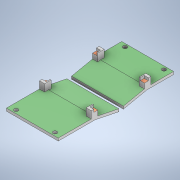
# Autodesk Inventor part: air_duct_inside
Saved by Autodesk Inventor 2022 (Build 260153000, 153)
## iProperties
Created: 2022-10-27
Part Number: air_duct_inside
Material: Ogólny
Document SubType Name: Modeling
Designer: kosak
Density: 1 g/cm^3
Appearance: Domyślna
Author: kosak
Autodesk Inventor part; units mm, degrees
ref_plane "YZ Plane" through (0, 0, 0) normal (1, 0, 0) x (0, 1, 0)
ref_plane "XZ Plane" through (0, 0, 0) normal (0, 1, 0) x (-1, 0, 0)
ref_plane "XY Plane" through (0, 0, 0) normal (0, 0, 1) x (1, 0, 0)
sketch "Szkic1" plane through (0, 0, 0) normal (0, 1, 0) x (-1, 0, 0)
  line L0 (0, 0) -> (40, 0)
  line L1 (40, 0) -> (40, -28.5)
  line L2 (40, -28.5) -> (0, -28.5)
  line L3 (0, -28.5) -> (0, 0)
  line L4 (0, -68.5) -> (40, -68.5)
  line L5 (40, -68.5) -> (40, -89)
  line L6 (40, -89) -> (0, -89)
  line L7 (0, -89) -> (0, -68.5)
  line L8 (22.9187, -28.5) -> (22.9187, -68.5)
  dimension "d0" = 40
  dimension "d1" = 28.5
  dimension "d3" = 20.5
  dimension "d84" = 40
  constraints: 18 end point, 4 parallel, 3 perpendicular, 2 horizontal, 2 point on line
  measures "d0" distance of L1.end L2.end
  measures "d1" distance of L0.end L1.end
  measures "d3" distance of L4.end L5.end
  measures "d84" distance of L8.start L8.end
extrude "Wyciągnięcie proste1" add sketch "Szkic1" along normal blind 2
sketch "Szkic2" plane through (0, 0, 0) normal (1, 0, 0) x (0, 0, -1)
  line L0 (48.4992, 0) -> (48.4992, -3.8)
  line L1 (0, 0) -> (28.5, 0) projected
  line L2 (28.5, 0) -> (48.5, 0)
  line L3 (89, 0) -> (68.5, 0) projected
  line L4 (48.4992, -3.8) -> (50.2492, -3.8)
  line L5 (48.4992, -3.8) -> (46.7492, -3.8)
  line L6 (28.5, 0) -> (46.7492, -3.8)
  line L7 (28.5, 0) -> (28.5, 2) projected
  line L8 (28.5, 2) -> (46.7492, -1.8)
  line L9 (46.7492, -1.8) -> (46.7492, -3.8)
  line L10 (68.5, 0) -> (50.2492, -3.8)
  line L11 (68.5, 0) -> (68.5, 2) projected
  line L12 (68.5, 2) -> (50.2492, -1.8)
  line L13 (50.2492, -1.8) -> (50.2492, -3.8)
  dimension "d8" = 20
  constraints: 20 end point, 4 parallel, 2 horizontal, 1 collinear, 1 point on line, 1 vertical
  measures "d8" distance of L1.end L2.end
extrude "Wyciągnięcie proste2" add sketch "Szkic2" against normal blind 40 contours L13 L12 L11 L10 | L8 L9 L6 L2 | L2 L7 L8
sketch "Szkic3" plane through (0, 2, 0) normal (0, 1, 0) x (1, 0, 0)
  line L0 (-40, 46.7492) -> (-40, 28.5) projected
  line L1 (-40, 28.5) -> (-36, 28.5)
  line L2 (-36, 28.5) -> (-36, 25.5)
  line L3 (-36, 25.5) -> (-40, 25.5)
  line L4 (-40, 25.5) -> (-40, 28.5)
  line L5 (-36, 28.5) -> (-40, 28.5)
  line L6 (-40, 28.5) -> (-40, 30.5)
  line L7 (-40, 30.5) -> (-36, 30.5)
  line L8 (-36, 30.5) -> (-36, 28.5)
  line L9 (-36, 71.5) -> (-36, 69.5)
  line L10 (-40, 71.5) -> (-36, 71.5)
  line L11 (-40, 69.5) -> (-40, 71.5)
  line L12 (-40, 66.5) -> (-40, 69.5)
  line L13 (-36, 66.5) -> (-40, 66.5)
  line L14 (-36, 69.5) -> (-36, 66.5)
  line L15 (0, 28.5) -> (0, 25.5)
  line L16 (0, 30.5) -> (0, 28.5)
  line L17 (-4, 30.5) -> (0, 30.5)
  line L18 (-4, 28.5) -> (-4, 30.5)
  line L19 (-4, 25.5) -> (-4, 28.5)
  line L20 (0, 25.5) -> (-4, 25.5)
  line L21 (-4, 71.5) -> (0, 71.5)
  line L22 (-4, 69.5) -> (-4, 71.5)
  line L23 (-4, 66.5) -> (-4, 69.5)
  line L24 (0, 69.5) -> (0, 66.5)
  line L25 (0, 71.5) -> (0, 69.5)
  line L26 (0, 66.5) -> (-4, 66.5)
  point P0 (0, 0)
  dimension "d13" = 4
  dimension "d14" = 3
  dimension "d15" = 2
  dimension "d18" = 41
  dimension "d25" = 36
  dimension "d32" = 36
  constraints: 52 end point, 4 horizontal, 4 parallel, 3 collinear, 2 perpendicular, 1 point on line, 1 vertical, 36 other
  measures "d13" distance of L2.end L3.end
  measures "d14" distance of L1.end L2.end
  measures "d15" distance of L5.end L6.end
  measures "d18" distance of L7.end L9.start
  measures "d25" distance of L1.end L15.start
  measures "d32" distance of L10.start L21.start
extrude "Wyciągnięcie proste3" add sketch "Szkic3" along normal blind 3.5
sketch "Szkic5" plane through (-40, 0, -89) normal (-1, 0, 0) x (0, 0, 1)
  line L0 (22.5, 2) -> (20.5, 2) projected
  line L1 (22.5, 2) -> (20.5, 2)
  line L2 (20.5, 2) -> (22.5, 1.5836)
  line L3 (38.7508, -1.8) -> (20.5, 2) projected
  line L4 (20.5, 2) -> (22.5, 2) projected
  line L5 (22.5, 2) -> (22.5, 1.5836)
  line L6 (58.5, 2) -> (60.5, 2) projected
  line L7 (60.5, 2) -> (42.2508, -1.8) projected
  line L8 (60.5, 2) -> (58.5, 2)
  line L9 (58.5, 1.5835) -> (58.5, 2)
  line L10 (58.5, 1.5835) -> (60.5, 2)
  point P0 (89, 0)
  constraints: 12 end point, 3 collinear, 2 perpendicular, 2 point on line
extrude "Wyciągnięcie proste5" add sketch "Szkic5" against normal blind 4
sketch "Szkic6" plane through (0, 5.5, 0) normal (0, 1, 0) x (1, 0, 0)
  line L0 (-36, 25.5) -> (-36, 30.5) projected
  line L1 (-36, 25.5) -> (-40, 25.5) projected
  line L2 (-36, 30.5) -> (-36.8, 30.5)
  line L3 (-36.8, 30.5) -> (-36.8, 25.5)
  line L4 (-36.8, 25.5) -> (-36, 25.5)
  line L5 (-36, 25.5) -> (-36, 30.5)
  line L6 (-36, 66.5) -> (-36, 71.5)
  line L7 (-36.8, 71.5) -> (-36.8, 66.5)
  line L8 (-36.8, 66.5) -> (-36, 66.5)
  line L9 (-36, 71.5) -> (-36.8, 71.5)
  line L10 (-4, 30.5) -> (-4, 25.5)
  line L11 (-3.2, 25.5) -> (-3.2, 30.5)
  line L12 (-3.2, 30.5) -> (-4, 30.5)
  line L13 (-4, 25.5) -> (-3.2, 25.5)
  line L14 (-4, 71.5) -> (-4, 66.5)
  line L15 (-3.2, 66.5) -> (-3.2, 71.5)
  line L16 (-3.2, 71.5) -> (-4, 71.5)
  line L17 (-4, 66.5) -> (-3.2, 66.5)
  point P0 (0, 0)
  dimension "d43" = 0.8
  dimension "d48" = 41
  dimension "d55" = 32.8
  constraints: 32 end point, 2 horizontal, 2 parallel, 1 collinear, 1 perpendicular, 1 point on line, 1 vertical, 24 other
  measures "d43" distance of L4.end L3.end
  measures "d48" distance of L4.end L6.start
  measures "d55" distance of L2.end L10.start
extrude "Wyciągnięcie proste6" add sketch "Szkic6" along normal blind 2
sketch "Szkic7" plane through (0, 5.5, 0) normal (0, 1, 0) x (1, 0, 0)
  line L0 (-40, 25.5) -> (-40, 0) projected
  line L1 (-36.8, 30.5) -> (-36.8, 25.5) projected
  line L2 (-40, 25.5) -> (-36.8, 25.5)
  line L3 (-36.8, 25.5) -> (-36.8, 27.5)
  line L4 (-36.8, 27.5) -> (-40, 27.5)
  line L5 (-40, 27.5) -> (-40, 25.5)
  line L6 (-36.8, 71.5) -> (-40, 71.5)
  line L7 (-40, 71.5) -> (-40, 69.5)
  line L8 (-40, 69.5) -> (-36.8, 69.5)
  line L9 (-36.8, 69.5) -> (-36.8, 71.5)
  line L10 (-3.2, 71.5) -> (-3.2, 69.5)
  line L11 (-3.2, 69.5) -> (0, 69.5)
  line L12 (0, 69.5) -> (0, 71.5)
  line L13 (0, 71.5) -> (-3.2, 71.5)
  line L14 (-3.2, 25.5) -> (0, 25.5)
  line L15 (-3.2, 27.5) -> (-3.2, 25.5)
  line L16 (0, 27.5) -> (-3.2, 27.5)
  line L17 (0, 25.5) -> (0, 27.5)
  point P0 (0, 0)
  dimension "d60" = 2
  dimension "d63" = 44
  dimension "d70" = 36.8
  dimension "d77" = 44
  constraints: 32 end point, 3 collinear, 2 horizontal, 2 parallel, 2 vertical, 1 perpendicular, 1 point on line, 21 other
  measures "d60" distance of L3.end L2.end
  measures "d63" distance of L3.end L6.start
  measures "d70" distance of L6.end L10.start
  measures "d77" distance of L10.end L14.start
extrude "Wyciągnięcie proste7" add sketch "Szkic7" along normal blind 2
sketch "Szkic8" plane through (0, 0, 0) normal (1, 0, 0) x (0, 0, -1)
  line L0 (28.5, 2) -> (30.5, 2) projected
  line L1 (28.5, 2) -> (30.5, 2)
  line L2 (30.5, 2) -> (30.5, 1.5835)
  line L3 (46.7492, -1.8) -> (28.5, 2) projected
  line L4 (28.5, 2) -> (30.5, 1.5835)
  line L5 (66.5, 2) -> (68.5, 2) projected
  line L6 (66.5, 2) -> (68.5, 2)
  line L7 (68.5, 2) -> (50.2492, -1.8) projected
  line L8 (66.5, 2) -> (66.5, 1.5836)
  line L9 (66.5, 1.5836) -> (68.5, 2)
  point P0 (0, 0)
  constraints: 12 end point, 2 collinear, 2 point on line, 1 horizontal, 1 perpendicular, 1 vertical
extrude "Wyciągnięcie proste8" add sketch "Szkic8" against normal blind 4
sketch "Szkic9" plane through (0, 2, 0) normal (0, 1, 0) x (1, 0, 0)
  line L0 (0, 0) -> (0, 25.5) projected
  line L1 (0, 2.5) -> (-5, 2.5)
  line L2 (-40, 0) -> (0, 0) projected
  line L3 (-5, 0) -> (-5, 2.5)
  line L4 (-40, 2.5) -> (-35, 2.5)
  line L5 (-35, 0) -> (-35, 2.5)
  circle A0 centre (-35, 2.5) radius 1.5
  circle A1 centre (-5, 2.5) radius 1.5
  circle A2 centre (-5, 86.5) radius 1.5
  circle A3 centre (-35, 86.5) radius 1.5
  dimension "d87" = 5
  dimension "d88" = 2.5
  dimension "d89" = 5
  dimension "d91" = 2.5
  dimension "d92" = 3
  dimension "d93" = 3
  dimension "d96" = 84
  constraints: 8 end point, 4 centre point, 3 point on line, 3 vertical, 2 coincident, 2 horizontal, 4 other
  measures "d87" distance of L1.start L1.end
  measures "d88" distance of L1.end L3.start
  measures "d89" distance of L4.end L4.start
  measures "d91" distance of L5.start L4.end
  measures "d92" diameter of A0
  measures "d93" diameter of A1
  measures "d96" distance of A1.centre A2.centre
extrude "Wyciągnięcie proste9" cut sketch "Szkic9" against normal blind 3 contours A0 L4 L5 | L5 L4 A0 | A1 L3 L1 | L1 L3 A1 | A2 | A3
equation "\"d101\" = d93"
